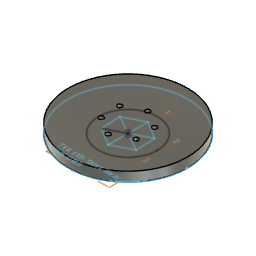
hexagon (Autodesk Fusion 360 design; units mm, degrees)
Autodesk Fusion 360 part; units mm, degrees
note: some values were not read from the file. Set by a fixed rule: the direction of a hole.
sketch "Sketch1" plane through (0, 0, 0) normal (0, 0, 1) x (1, 0, 0)
  circle A0 centre (0, 0) radius 6.35
  line L0 (3.2944, -2.3723) -> (3.6944, -2.3672) construction
  line L1 (3.6944, -2.3672) -> (3.6801, -1.2492) construction
  line L2 (3.6801, -1.2492) -> (3.2802, -1.2543) construction
  line L3 (3.2802, -1.2543) -> (3.2944, -2.3723) construction
  line L4 (3.1438, 0.9835) -> (3.5438, 0.9886) construction
  line L5 (3.5438, 0.9886) -> (3.5296, 2.1067) construction
  line L6 (3.5296, 2.1067) -> (3.1296, 2.1016) construction
  line L7 (3.1296, 2.1016) -> (3.1438, 0.9835) construction
  line L8 (0.0593, 3.16) -> (0.4593, 3.1651) construction
  line L9 (0.4593, 3.1651) -> (0.445, 4.2832) construction
  line L10 (0.445, 4.2832) -> (0.0451, 4.2781) construction
  line L11 (0.0451, 4.2781) -> (0.0593, 3.16) construction
  line L12 (0, 0) -> (0, 2.112)
  line L13 (0, 0) -> (1.8752, 0.9629)
  line L14 (0, 0) -> (1.9668, -1.101)
  line L15 (0, 0) -> (-0.0074, -2.108)
  line L16 (0, 0) -> (-1.8821, -0.9582)
  line L17 (0, 0) -> (-1.9753, 1.1062)
  line L18 (0, 2.112) -> (1.8752, 0.9629)
  line L19 (1.8752, 0.9629) -> (1.9668, -1.101)
  line L20 (1.9668, -1.101) -> (-0.0074, -2.108)
  line L21 (-0.0074, -2.108) -> (-1.8821, -0.9582)
  line L22 (-1.8821, -0.9582) -> (-1.9753, 1.1062)
  line L23 (-1.9753, 1.1062) -> (0, 2.112)
  line L24 (-2.6701, -6.0055) -> (3.9819, -6.0007) construction
  line L25 (3.9819, -6.0007) -> (3.9807, -4.3891) construction
  line L26 (3.9807, -4.3891) -> (-2.6712, -4.3939) construction
  line L27 (-2.6712, -4.3939) -> (-2.6701, -6.0055) construction
  circle A1 centre (0, 0) radius 3.12
  dimension "d7" = 12.7
  dimension "d18" = 2.112
  dimension "d19" = 2.108
  dimension "d20" = 62.82
  dimension "d21" = 2.254
  dimension "d22" = 119.24
  dimension "d23" = 2.108
  dimension "d24" = 180.2
  dimension "d25" = 2.112
  dimension "d26" = 116.98
  dimension "d27" = 2.264
  dimension "d28" = 60.75
  dimension "d29" = 6.24
  constraint coincident A0.centre L12.start
  constraint vertical L12
  measures "d7" diameter of A0
  measures "d18" distance of A0.centre L12.end
  measures "d19" distance of A0.centre L13.end
  measures "d20" angle of L12 L13
  measures "d21" distance of A0.centre L14.end
  measures "d22" angle of L12 L14
  measures "d23" vertical distance of A0.centre L15.end
  measures "d25" distance of A0.centre L16.end
  measures "d26" angle of L12 L16
  measures "d27" distance of A0.centre L17.end
  measures "d28" angle of L12 L17
  measures "d29" diameter of A1
extrude "Extrude2" add sketch "Sketch1" along normal blind 1 contours A0 | L12 L17 L23 | L12 L13 L18 | L13 L14 L19 | L14 L15 L20 | L15 L16 L21 | L16 L17 L22 | A1
hole "Hole2" at (0, 2.112, 0) at (1.8752, 0.9629, 0) at (1.9668, -1.101, 0) at (-0.0074, -2.108, 0) at (-1.8821, -0.9582, 0) at (-1.9753, 1.1062, 0) direction (0, 0, 1) diameter 0.5 depth 1 tip angle 118
equation "d26 = 360 deg - 243.02 deg"
equation "d28 = 360 deg - 299.25 deg"
